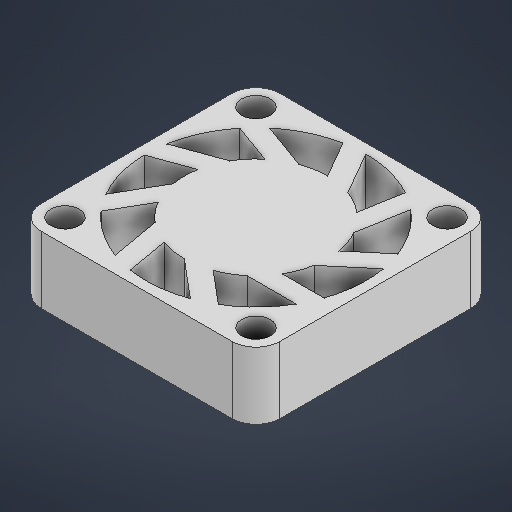
# Autodesk Inventor part: Fan
Saved by Autodesk Inventor 2026.1 (Build 301233020, 233B)
## iProperties
Created: 2026-03-17
Part Number: Fan
Material: 一般
Document SubType Name: Modeling
Designer: kamada
Density: 1 g/cm^3
Appearance: 既定
Author: kamada
Autodesk Inventor part; units mm, degrees
ref_plane "YZ Plane" through (0, 0, 0) normal (1, 0, 0) x (0, 1, 0)
ref_plane "XZ Plane" through (0, 0, 0) normal (0, 1, 0) x (-1, 0, 0)
ref_plane "XY Plane" through (0, 0, 0) normal (0, 0, 1) x (1, 0, 0)
sketch "スケッチ1" plane through (0, 0, 0) normal (0, 1, 0) x (-1, 0, 0)
  line L0 (12.5, 12.5) -> (-12.5, 12.5)
  line L1 (-12.5, 12.5) -> (-12.5, -12.5)
  line L2 (-12.5, -12.5) -> (12.5, -12.5)
  line L3 (12.5, -12.5) -> (12.5, 12.5)
  line L4 (10, -10) -> (-10, -10)
  line L5 (-10, -10) -> (-10, 10)
  line L6 (-10, 10) -> (10, 10)
  line L7 (10, 10) -> (10, -10)
  circle A0 centre (10, -10) radius 1.5
  circle A1 centre (-10, -10) radius 1.5
  circle A2 centre (-10, 10) radius 1.5
  circle A3 centre (10, 10) radius 1.5
  circle A4 centre (10, 10) radius 2.5
  circle A5 centre (-10, 10) radius 2.5
  circle A6 centre (-10, -10) radius 2.5
  circle A7 centre (10, -10) radius 2.5
  circle A8 centre (0, 0) radius 11.5
  circle A9 centre (0, 0) radius 7.5
  point P0 (12.5, 0)
  point P1 (0, -12.5)
  point P2 (-10, 0)
  point P3 (-12.5, 0)
  point P4 (0, -10)
  point P5 (12.5, 10)
  point P6 (10, 12.5)
  point P7 (-10, 12.5)
  point P8 (-12.5, 10)
  point P9 (-12.5, -10)
  point P10 (-10, -12.5)
  point P11 (10, -12.5)
  point P12 (12.5, -10)
  point P13 (-5.6789, 10)
  point P14 (5.6789, 10)
  dimension "d0" = 25
  dimension "d1" = 25
  dimension "d2" = 20
  dimension "d3" = 20
  dimension "d4" = 3
  dimension "d5" = 3
  dimension "d6" = 3
  dimension "d7" = 3
  dimension "d8" = 23
  dimension "d9" = 15
  constraints: 16 end point, 10 centre point, 10 coincident, 5 midpoint, 4 parallel, 2 horizontal, 2 horizontal alignment, 2 perpendicular, 2 tangent, 2 vertical alignment
  measures "d0" distance of L2.end L1.end
  measures "d1" distance of L1.end L0.end
  measures "d2" distance of L5.end L6.end
  measures "d3" distance of L4.end L5.end
  measures "d4" diameter of A0
  measures "d5" diameter of A1
  measures "d6" diameter of A2
  measures "d7" diameter of A3
  measures "d8" diameter of A8
  measures "d9" diameter of A9
extrude "押し出し1" add sketch "スケッチ1" along normal blind 7 contours A4 L6 A8 A5 L0 | A4 L7 A3 L6 | L3 A7 L7 A8 A4 | A5 L6 A2 L5 | A4 L7 A8 L6 | L6 A3 L7 A4 | A7 L4 A0 L7 | A5 L5 A2 L6 | L6 A8 L5 A5 | A5 L5 A8 A6 L1 | A7 L4 A8 L7 | L7 A0 L4 A7 | L2 A6 L4 A8 A7 | A6 L5 A1 L4 | A6 L4 A1 L5 | L5 A8 L4 A6 | A9
sketch "スケッチ2" plane through (0, 7, 0) normal (0, 1, 0) x (1, 0, 0)
  circle A0 centre (0, 0) radius 7.5 projected
  circle A1 centre (0, 0) radius 11.5 projected
  line L0 (0, 7.5) -> (-2.1881, 11.2899)
  line L1 (0, 7.5) -> (4.3762, 7.5) construction
  line L2 (0, 11.5) -> (3.4783, 5.4754)
  line L3 (0, 11.5) -> (6.9566, 11.5) construction
  line L4 (-4.8209, 5.7453) -> (-8.9332, 7.2421)
  line L5 (-7.3921, 8.8095) -> (-0.855, 6.4302)
  line L6 (-7.3861, 1.3024) -> (-11.4984, -0.1944)
  line L7 (-11.3253, 1.997) -> (-4.7882, 4.3763)
  line L8 (-6.4952, -3.75) -> (-8.6833, -7.5399)
  line L9 (-9.9593, -5.75) -> (-6.481, 0.2746)
  line L10 (-2.5652, -7.0477) -> (-1.8052, -11.3574)
  line L11 (-3.9332, -10.8065) -> (-5.1412, -3.9555)
  line L12 (2.5652, -7.0477) -> (5.9175, -9.8607)
  line L13 (3.9332, -10.8065) -> (-1.3958, -6.3348)
  line L14 (6.4952, -3.75) -> (10.8714, -3.75)
  line L15 (9.9593, -5.75) -> (3.0027, -5.75)
  line L16 (7.3861, 1.3024) -> (10.7384, 4.1153)
  line L17 (11.3253, 1.997) -> (5.9962, -2.4747)
  line L18 (4.8209, 5.7453) -> (5.5808, 10.0551)
  line L19 (7.3921, 8.8095) -> (6.1841, 1.9586)
  point P0 (-2.5583, 7.0502)
  point P1 (-6.4916, 3.7563)
  point P2 (-7.3873, -1.2952)
  point P3 (-4.8265, -5.7407)
  point P4 (-0.0073, -7.5)
  point P5 (4.8153, -5.75)
  point P6 (7.3848, -1.3095)
  point P7 (6.4988, 3.7437)
  point P8 (2.572, 7.0452)
  dimension "d12" = 120
  dimension "d13" = 60
  dimension "d16" = 360
  constraints: 40 end point, 2 equal length, 2 horizontal, 2 point on circle, 57 other
  measures "d12" angle of L1 L0
  measures "d13" angle of L2 L3
extrude "押し出し2" add sketch "スケッチ2" against normal up to surface (7 mm away) contours A0 L16 A1 L17 | A0 L18 A1 L19 | L14 A1 L15 A0 | A0 L0 A1 L2 | L12 A1 L13 A0 | A0 L4 A1 L5 | L10 A1 L11 A0 | A0 L6 A1 L7 | L8 A1 L9 A0
